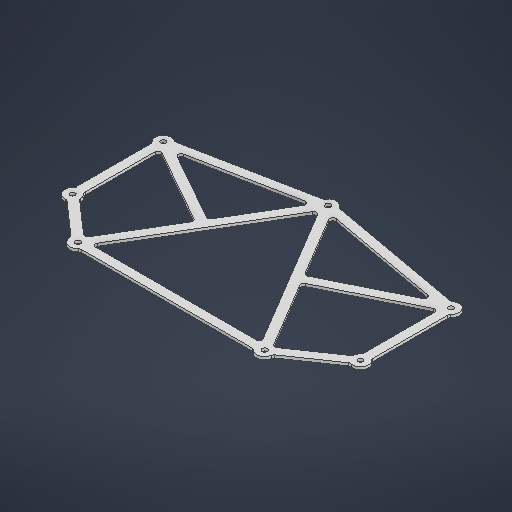
# Autodesk Inventor part: bed-interface
Saved by Autodesk Inventor 2025 (Build 290162000, 162)
## iProperties
Created: 2024-07-18
Part Number: bed-interface
Material: Generic
Document SubType Name: Sheet Metal
Designer: Windows 7 was better
Density: 1 g/cm^3
Appearance: Default
Sheet Metal Rule: Default
Author: Windows 7 was better
Autodesk Inventor part; units mm, degrees
ref_plane "YZ Plane" through (0, 0, 0) normal (1, 0, 0) x (0, 1, 0)
ref_plane "XZ Plane" through (0, 0, 0) normal (0, 1, 0) x (-1, 0, 0)
ref_plane "XY Plane" through (0, 0, 0) normal (0, 0, 1) x (1, 0, 0)
sketch "Sketch1" plane through (0, 0, 0) normal (0, 1, 0) x (-1, 0, 0)
  line L0 (-156.8414, -221.8409) -> (143.1586, -221.8409) construction
  line L1 (0, -221.8409) -> (0, -201.8409) construction
  circle A0 centre (0, -201.8409) radius 3
  line L2 (0, -201.8409) -> (103.0047, -28.8431) construction
  line L3 (0, -201.8409) -> (201.341, -201.8409) construction
  line L4 (103.0047, -28.8431) -> (-102.9953, -28.8431) construction
  circle A1 centre (103.0047, -28.8431) radius 3
  circle A2 centre (-102.9953, -28.8431) radius 3
  circle A3 centre (0, -201.8409) radius 9
  circle A4 centre (103.0047, -28.8431) radius 9
  circle A5 centre (-102.9953, -28.8431) radius 9
  circle A6 centre (151.9636, -171.8409) radius 2.805 construction
  circle A7 centre (151.9636, -71.8409) radius 2.805 construction
  circle A8 centre (-165.6464, -71.8409) radius 2.805 construction
  circle A9 centre (-165.6464, -171.8409) radius 2.805 construction
  line L5 (151.9636, -171.8409) -> (151.9636, -71.8409) construction
  line L6 (151.9636, -71.8409) -> (103.0047, -28.8431) construction
  line L7 (151.9636, -171.8409) -> (0, -201.8409) construction
  line L8 (0, -201.8409) -> (-165.6464, -171.8409) construction
  line L9 (-165.6464, -171.8409) -> (-165.6464, -71.8409) construction
  line L10 (-165.6464, -71.8409) -> (-102.9953, -28.8431) construction
  line L11 (-102.9953, -28.8431) -> (0, -201.8409) construction
  line L12 (151.9636, -171.8409) -> (51.5023, -115.342) construction
  line L13 (-51.4977, -115.342) -> (-165.6464, -171.8409) construction
  line L14 (49.0514, -119.7001) -> (149.5126, -176.199)
  line L15 (149.5126, -176.199) -> (154.4145, -167.4829)
  line L16 (154.4145, -167.4829) -> (53.9533, -110.984)
  line L17 (53.9533, -110.984) -> (49.0514, -119.7001)
  line L18 (49.0514, -119.7001) -> (154.4145, -167.4829) construction
  line L19 (149.5126, -176.199) -> (53.9533, -110.984) construction
  line L20 (4.2961, -204.3989) -> (107.3008, -31.4011)
  line L21 (107.3008, -31.4011) -> (98.7085, -26.2852)
  line L22 (98.7085, -26.2852) -> (-4.2961, -199.283)
  line L23 (-4.2961, -199.283) -> (4.2961, -204.3989)
  line L24 (4.2961, -204.3989) -> (98.7085, -26.2852) construction
  line L25 (107.3008, -31.4011) -> (-4.2961, -199.283) construction
  line L26 (-4.2962, -204.3987) -> (-107.2916, -31.4009)
  line L27 (-107.2916, -31.4009) -> (-98.6991, -26.2853)
  line L28 (-98.6991, -26.2853) -> (4.2962, -199.2831)
  line L29 (4.2962, -199.2831) -> (-4.2962, -204.3987)
  line L30 (-4.2962, -204.3987) -> (-98.6991, -26.2853) construction
  line L31 (-107.2916, -31.4009) -> (4.2962, -199.2831) construction
  line L32 (-163.4285, -176.3221) -> (-49.2797, -119.8232)
  line L33 (-49.2797, -119.8232) -> (-53.7156, -110.8609)
  line L34 (-53.7156, -110.8609) -> (-167.8644, -167.3598)
  line L35 (-167.8644, -167.3598) -> (-163.4285, -176.3221)
  line L36 (-163.4285, -176.3221) -> (-53.7156, -110.8609) construction
  line L37 (-49.2797, -119.8232) -> (-167.8644, -167.3598) construction
  line L38 (103.0047, -33.8431) -> (-102.9953, -33.8431)
  line L39 (-102.9953, -33.8431) -> (-102.9953, -23.8431)
  line L40 (-102.9953, -23.8431) -> (103.0047, -23.8431)
  line L41 (103.0047, -23.8431) -> (103.0047, -33.8431)
  line L42 (103.0047, -33.8431) -> (-102.9953, -23.8431) construction
  line L43 (-102.9953, -33.8431) -> (103.0047, -23.8431) construction
  line L44 (-162.8171, -75.9634) -> (-100.166, -32.9656)
  line L45 (-100.166, -32.9656) -> (-105.8246, -24.7206)
  line L46 (-105.8246, -24.7206) -> (-168.4757, -67.7184)
  line L47 (-168.4757, -67.7184) -> (-162.8171, -75.9634)
  line L48 (-162.8171, -75.9634) -> (-105.8246, -24.7206) construction
  line L49 (-100.166, -32.9656) -> (-168.4757, -67.7184) construction
  circle A10 centre (-165.6464, -71.8409) radius 2.805
  circle A11 centre (-165.6464, -71.8409) radius 8.805
  circle A12 centre (-165.6464, -171.8409) radius 2.805
  circle A13 centre (-165.6464, -171.8409) radius 8.805
  circle A14 centre (151.9636, -171.8409) radius 2.805
  circle A15 centre (151.9636, -171.8409) radius 8.805
  circle A16 centre (151.9636, -71.8409) radius 2.805
  circle A17 centre (151.9636, -71.8409) radius 8.805
  line L50 (-160.6464, -171.8409) -> (-160.6464, -71.8409)
  line L51 (-160.6464, -71.8409) -> (-170.6464, -71.8409)
  line L52 (-170.6464, -71.8409) -> (-170.6464, -171.8409)
  line L53 (-170.6464, -171.8409) -> (-160.6464, -171.8409)
  line L54 (-160.6464, -171.8409) -> (-170.6464, -71.8409) construction
  line L55 (-160.6464, -71.8409) -> (-170.6464, -171.8409) construction
  line L56 (-0.891, -206.7609) -> (-166.5375, -176.7609)
  line L57 (-166.5375, -176.7609) -> (-164.7554, -166.921)
  line L58 (-164.7554, -166.921) -> (0.891, -196.921)
  line L59 (0.891, -196.921) -> (-0.891, -206.7609)
  line L60 (-0.891, -206.7609) -> (-164.7554, -166.921) construction
  line L61 (-166.5375, -176.7609) -> (0.891, -196.921) construction
  line L62 (0.9684, -206.7463) -> (152.9319, -176.7463)
  line L63 (152.9319, -176.7463) -> (150.9952, -166.9356)
  line L64 (150.9952, -166.9356) -> (-0.9684, -196.9356)
  line L65 (-0.9684, -196.9356) -> (0.9684, -206.7463)
  line L66 (0.9684, -206.7463) -> (150.9952, -166.9356) construction
  line L67 (152.9319, -176.7463) -> (-0.9684, -196.9356) construction
  line L68 (146.9636, -171.8409) -> (146.9636, -71.8409)
  line L69 (146.9636, -71.8409) -> (156.9636, -71.8409)
  line L70 (156.9636, -71.8409) -> (156.9636, -171.8409)
  line L71 (156.9636, -171.8409) -> (146.9636, -171.8409)
  line L72 (146.9636, -171.8409) -> (156.9636, -71.8409) construction
  line L73 (146.9636, -71.8409) -> (156.9636, -171.8409) construction
  line L74 (99.7052, -32.6) -> (148.6641, -75.5978)
  line L75 (148.6641, -75.5978) -> (155.263, -68.0841)
  line L76 (155.263, -68.0841) -> (106.3041, -25.0863)
  line L77 (106.3041, -25.0863) -> (99.7052, -32.6)
  line L78 (99.7052, -32.6) -> (155.263, -68.0841) construction
  line L79 (148.6641, -75.5978) -> (106.3041, -25.0863) construction
  point P0 (0, 0)
  point P1 (101.7329, -143.5915)
  point P2 (-108.5721, -143.5915)
  point P3 (0.0047, -28.8431)
  point P4 (-134.3209, -50.342)
  point P5 (-165.6464, -121.8409)
  point P6 (-82.8232, -186.8409)
  point P7 (75.9818, -186.8409)
  point P8 (151.9636, -121.8409)
  point P9 (127.4841, -50.342)
  point P10 (-94.1995, -33.8431)
  point P11 (94.2084, -33.8431)
  point P12 (0.0002, -192.0672)
  point P13 (-166.8907, -169.327)
  point P14 (-164.4022, -174.3549)
  point P15 (143.2185, -70.8152)
  point P16 (146.9636, -79.0886)
  point P17 (146.9636, -163.2925)
  point P18 (58.4205, -113.4963)
  point P19 (103.4724, -37.831)
  point P20 (105.328, -37.5381)
  point P21 (10.033, -194.7638)
  point P22 (53.303, -122.0912)
  point P23 (137.7061, -169.5591)
  point P24 (-149.8784, -169.6153)
  point P25 (-53.4268, -121.8758)
  point P26 (-9.9131, -194.9642)
  point P27 (-106.336, -37.2001)
  point P28 (-103.4634, -37.831)
  point P29 (-58.5577, -113.2575)
  point P30 (-160.6464, -163.7872)
  point P31 (-160.6464, -79.0886)
  point P32 (-156.8415, -71.8623)
  point P33 (-95.512, -23.8431)
  point P34 (-111.9946, -28.9551)
  point P35 (-162.5001, -63.6173)
  point P36 (-170.6464, -79.0886)
  point P37 (-170.6464, -164.5933)
  point P38 (-159.4059, -178.0525)
  point P39 (-8.2546, -205.4273)
  point P40 (8.31, -205.2969)
  point P41 (145.8216, -178.15)
  point P42 (156.9636, -164.5933)
  point P43 (156.9636, -79.0886)
  point P44 (149.8173, -63.3015)
  point P45 (111.9268, -30.0244)
  point P46 (95.5213, -23.8431)
  dimension "d0" = 20
  dimension "d1" = 6
  dimension "d2" = 201.341
  dimension "d3" = 59.23
  dimension "d4" = 206
  dimension "d5" = 6
  dimension "d6" = 6
  dimension "d7" = 6
  dimension "d8" = 6
  dimension "d9" = 6
  dimension "d10" = 10
  dimension "d11" = 10
  dimension "d12" = 10
  dimension "d13" = 10
  dimension "d14" = 10
  dimension "d15" = 10
  dimension "d16" = 6
  dimension "d17" = 6
  dimension "d18" = 6
  dimension "d19" = 6
  dimension "d20" = 10
  dimension "d21" = 10
  dimension "d22" = 10
  dimension "d23" = 10
  dimension "d24" = 10
  measures "d0" distance of L1.start L1.end
  measures "d1" diameter of A0
  measures "d2" distance of L2.start L2.end
  measures "d3" angle of L3 L2
  measures "d4" distance of L2.end L4.end
  measures "d5" diameter of A1
  measures "d6" diameter of A2
  measures "d7" radial gap between concentric circles of A0 A3
  measures "d8" radial gap between concentric circles of A1 A4
  measures "d9" radial gap between concentric circles of A2 A5
  measures "d10" distance of L15.end L14.end
  measures "d11" distance of L21.end L20.end
  measures "d12" distance of L26.end L27.end
  measures "d13" distance of L33.end L32.end
  measures "d14" distance of L38.end L39.end
  measures "d15" distance of L45.end L44.end
  measures "d16" radial gap between concentric circles of A8 A11
  measures "d17" radial gap between concentric circles of A9 A13
  measures "d18" radial gap between concentric circles of A6 A15
  measures "d19" radial gap between concentric circles of A7 A17
  measures "d20" distance of L51.end L50.end
  measures "d21" distance of L56.end L57.end
  measures "d22" distance of L63.end L62.end
  measures "d23" distance of L68.end L69.end
  measures "d24" distance of L75.end L74.end
extrude "Plate1" add sketch "Sketch1" along normal blind 3.048 contours A0 L29 L28 L64 A3 L20 L23 | A0 L59 L58 L64 L28 L29 | L23 L20 A3 L62 L65 A0 | A0 L65 L64 L58 L59 | L65 L62 A3 L56 L59 A0 | A0 L23 L22 L58 L64 L65 | L64 L58 L22 A3 L28 | L28 A3 L64 | A0 L29 L26 A3 L58 L22 L23 | A0 L59 L56 A3 L26 L29 | L20 L64 L14 A15 L62 A3 | A3 L64 L20 | L28 L22 L38 A4 L20 L16 L17 L14 L64 A3 | A3 L22 L28 | L58 A3 L22 | A3 L58 L26 L32 L33 L34 A5 L38 L28 L22 | L26 L58 A3 | A3 L56 A13 L32 L58 L26 | L62 L63 A14 L71 L70 A15 | A15 L14 L15 A14 L63 L62 | L20 L16 L68 A15 L64 L14 | L14 L17 L16 L20 | L64 A15 L14 | L38 L28 A5 L40 A4 L22 | L22 A4 L38 | L38 A5 L28 | L56 L57 A12 L35 L32 A13 | A13 L52 L53 A12 L57 L56 | A15 L64 L68 L71 A14 L15 L14 | A15 L68 L64 | L22 L21 A1 L77 L74 L38 A4 | A4 L40 L41 A1 L21 L22 | L38 L74 L20 A4 | L28 L27 A2 L39 L40 A5 | A5 L38 L44 L45 A2 L27 L28 | A5 L26 L44 L38 | L32 L58 A13 L50 L34 L26 | L26 L34 L33 L32 | L32 A13 L58 | L52 A11 L50 L34 A13 | A13 L34 L35 A12 L53 L52 | L32 L35 A12 L53 L50 L58 A13 | L70 L71 A14 L15 L16 A15 | A15 L16 L68 A17 L70 | L16 A15 L68 | L20 L74 A4 | A15 L16 L15 A14 L63 L64 L68 | L64 L63 A14 L71 L68 | A4 L76 L77 A1 L41 L40 | L74 L77 A1 L41 L38 | L38 L41 A1 L21 L20 L74 | A5 L44 L26 | L44 L26 L27 A2 L39 L38 | L38 L39 A2 L45 L44 | L58 L50 A13 | A13 L50 L58 L57 A12 L35 L34 | L34 L50 A13 | L52 L51 A10 L47 L44 L50 A11 | A11 L46 L47 A10 L51 L52 | L70 L69 A16 L75 L76 A17 | A17 L68 L74 L75 A16 L69 L70 | A17 L74 L68 | L74 L20 L21 A1 L77 L76 A4 | A4 L76 A17 L74 | L40 L39 A2 L45 L46 A5 | L44 A11 L46 A5 | A5 L46 L45 A2 L27 L26 L44 | L50 L53 A12 L57 L58 | A11 L44 L50 L51 A10 L47 L46 | L50 L44 A11 | A17 L76 L75 A16 L69 L68 L74 | L68 L69 A16 L75 L74 | L44 L47 A10 L51 L50
fillet "Corner Round1" radius 3.175 35 edges at (58.5577, 1.524, -113.2575) (160.6464, 1.524, -163.7872) (160.6464, 1.524, -79.0886) (156.8415, 1.524, -71.8623) (106.336, 1.524, -37.2001) (103.4634, 1.524, -37.831) (-137.7061, 1.524, -169.5591) (-10.033, 1.524, -194.7638) (-53.303, 1.524, -122.0912) (-146.9636, 1.524, -163.2925) (-58.4205, 1.524, -113.4963) (-103.4724, 1.524, -37.831) (-105.328, 1.524, -37.5381) (-143.2185, 1.524, -70.8152) (-146.9636, 1.524, -79.0886) (9.9131, 1.524, -194.9642) (149.8784, 1.524, -169.6153) (53.4268, 1.524, -121.8758) (-0.0002, 1.524, -192.0672) (94.1995, 1.524, -33.8431) (-94.2084, 1.524, -33.8431) (95.512, 1.524, -23.8431) (111.9946, 1.524, -28.9551) (-95.5213, 1.524, -23.8431) (-111.9268, 1.524, -30.0244) (-149.8173, 1.524, -63.3015) (-156.9636, 1.524, -79.0886) (-156.9636, 1.524, -164.5933) (-145.8216, 1.524, -178.15) (-8.31, 1.524, -205.2969) (8.2546, 1.524, -205.4273) (159.4059, 1.524, -178.0525) (170.6464, 1.524, -164.5933) (170.6464, 1.524, -79.0886) (162.5001, 1.524, -63.6173)
body "Solid2"
